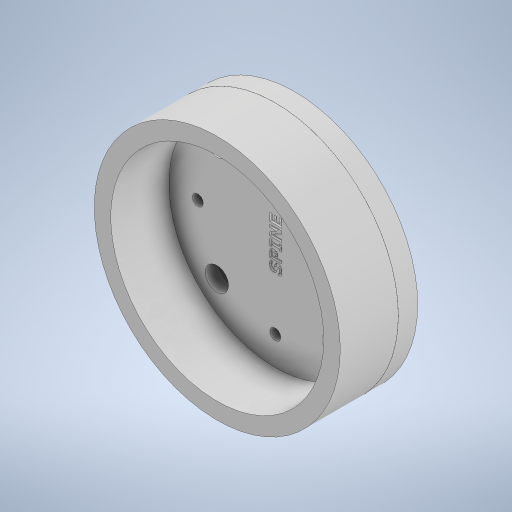
# Autodesk Inventor part: adaptor_spine_transducer_names
Saved by Autodesk Inventor 2024 (Build 280153000, 153)
## iProperties
Created: 2024-05-24
Part Number: adaptor_spine_transducer_names
Material: Generic
Document SubType Name: Modeling
Designer: maint
Density: 1 g/cm^3
Appearance: Default
Author: maint
Autodesk Inventor part; units mm, degrees
ref_plane "YZ Plane" through (0, 0, 0) normal (1, 0, 0) x (0, 1, 0)
ref_plane "XZ Plane" through (0, 0, 0) normal (0, 1, 0) x (-1, 0, 0)
ref_plane "XY Plane" through (0, 0, 0) normal (0, 0, 1) x (1, 0, 0)
sketch "Sketch1" plane through (0, 0, 0) normal (0, 0, 1) x (1, 0, 0)
  line L0 (40, -40) -> (-40, -40)
  line L1 (-40, -40) -> (-40, 40)
  line L2 (-40, 40) -> (40, 40)
  line L3 (40, 40) -> (40, -40)
  line L4 (40, -40) -> (-40, 40) construction
  line L5 (-40, -40) -> (40, 40) construction
  circle A0 centre (0, 0) radius 63.5
  dimension "d0" = 80
  dimension "d72" = 127
  constraints: 12 end point, 2 midpoint, 2 parallel, 2 perpendicular, 1 centre point, 1 coincident, 1 horizontal
  measures "d0" distance of L1.end L2.end
  measures "d72" diameter of A0
extrude "Extrusion1" add sketch "Sketch1" along normal blind 10 contours L0 L1 L2 L3 | A0
sketch "Sketch2" plane through (0, 0, 0) normal (0, 0, -1) x (-1, 0, 0)
  arc A0 (40, 37) -> (37, 40) centre (37, 37) ccw
  line L0 (30.15, -30.15) -> (-30.15, -30.15)
  line L1 (-30.15, -30.15) -> (-30.15, 30.15)
  line L2 (-30.15, 30.15) -> (30.15, 30.15)
  line L3 (30.15, 30.15) -> (30.15, -30.15)
  line L4 (30.15, -30.15) -> (-30.15, 30.15) construction
  line L5 (-30.15, -30.15) -> (30.15, 30.15) construction
  circle A1 centre (-30.15, 30.15) radius 4.75
  circle A2 centre (30.15, 30.15) radius 4.75
  circle A3 centre (30.15, -30.15) radius 4.75
  circle A4 centre (-30.15, -30.15) radius 4.75
  point P0 (0, 0)
  point P1 (39.1213, 39.1213)
  dimension "d32" = 60.3
  dimension "d33" = 9.5
  constraints: 12 end point, 5 centre point, 4 coincident, 3 equal radius, 3 point on circle, 2 midpoint, 2 parallel, 2 perpendicular, 1 horizontal
  measures "d32" distance of L1.end L2.end
  measures "d33" diameter of A2
hole "Hole3" at (30.15, -30.15, 0) at (30.15, 30.15, 0) at (-30.15, 30.15, 0) at (-30.15, -30.15, 0) direction (0, 0, 1) diameter 6.6 end through all
sketch "Sketch3" plane through (0, 0, 0) normal (0, 0, -1) x (-1, 0, 0)
  circle A0 centre (0, 0) radius 40
  circle A1 centre (0, 40) radius 2.5
  circle A2 centre (40, 0) radius 2.5
  circle A3 centre (0, -40) radius 2.5
  circle A4 centre (-40, 0) radius 2.5
  dimension "d12" = 5
  dimension "d60" = 80
  constraints: 5 centre point, 4 point on circle, 3 equal radius
  measures "d12" diameter of A1
  measures "d60" diameter of A0
hole "Hole1" at (40, 0, 0) at (0, 40, 0) at (0, -40, 0) at (-40, 0, 0) direction (0, 0, 1) diameter 5.6 end through all
sketch "Sketch8" plane through (0, 0, 0) normal (0, 0, -1) x (-1, 0, 0)
  circle A0 centre (0, 0) radius 40
  circle A1 centre (0, 40) radius 12.0233
  circle A2 centre (40, 0) radius 12.001
  circle A3 centre (-40, 0) radius 12.185
  circle A4 centre (0, -40) radius 12.001
  dimension "d61" = 80
  constraints: 5 centre point, 4 point on circle, 1 coincident
  measures "d61" diameter of A0
hole "Hole4" at (-40, 0, 0) at (0, 40, 0) at (40, 0, 0) at (0, -40, 0) direction (0, 0, 1) diameter 13 depth 4 tip angle 118
sketch "Sketch10" plane through (0, 0, 10) normal (0, 0, 1) x (1, 0, 0)
  circle A0 centre (30.15, 30.15) radius 3.3 projected
  circle A1 centre (30.15, 30.15) radius 6
  circle A2 centre (-30.15, 30.15) radius 3.3 projected
  circle A3 centre (-30.15, 30.15) radius 6
  circle A4 centre (-30.15, -30.2444) radius 6
  circle A5 centre (30.15, -30.2444) radius 6
  point P0 (0, 0)
  dimension "d63" = 12
  constraints: 4 centre point, 3 equal radius, 2 coincident
  measures "d63" diameter of A1
hole "Hole5" at (-30.15, -30.2444, 10) at (30.15, -30.2444, 10) at (30.15, 30.15, 10) at (-30.15, 30.15, 10) direction (0, 0, -1) diameter 12 depth 7 tip angle 118
sketch "Sketch11" plane through (0, 0, 0) normal (0, 0, -1) x (-1, 0, 0)
  line L0 (2.543, 18.4604) -> (2.543, -5.1802) construction
  line L1 (2.543, -5.1802) -> (11.8674, -5.1802) construction
  line L2 (11.8674, -5.1802) -> (11.8674, 18.4604) construction
  line L3 (11.8674, 18.4604) -> (2.543, 18.4604) construction
  spline S0 degree 2 poles (-3.7943, 15.9443) (-3.7943, 16.6463) (-3.5224, 17.7041) (-3.3246, 18.1589) knots 0 0 0 1 2 2 2
  line L4 (-3.3246, 18.1589) -> (-1.8713, 18.1589)
  line L5 (-1.8713, 18.1589) -> (-1.8713, 18.0205)
  spline S1 degree 2 poles (-1.8713, 18.0205) (-2.2618, 17.5608) (-2.682, 16.4584) (-2.682, 15.9394) knots 0 0 0 1 2 2 2
  spline S2 degree 2 poles (-2.682, 15.9394) (-2.682, 15.8059) (-2.6227, 15.3758) (-2.5634, 15.2473) knots 0 0 0 1 2 2 2
  spline S3 degree 2 poles (-2.5634, 15.2473) (-2.4942, 15.0891) (-2.2421, 14.8667) (-2.0394, 14.8667) knots 0 0 0 1 2 2 2
  spline S4 degree 2 poles (-2.0394, 14.8667) (-1.8071, 14.8667) (-1.5204, 15.2275) (-1.4561, 15.4747) knots 0 0 0 1 2 2 2
  spline S5 degree 2 poles (-1.4561, 15.4747) (-1.3721, 15.7861) (-1.2287, 16.493) (-1.1199, 16.8044) knots 0 0 0 1 2 2 2
  spline S6 degree 2 poles (-1.1199, 16.8044) (-0.8728, 17.5113) (-0.0275, 18.1243) (0.6053, 18.1243) knots 0 0 0 1 2 2 2
  spline S7 degree 2 poles (0.6053, 18.1243) (1.4604, 18.1243) (2.5232, 16.6759) (2.5232, 15.5884) knots 0 0 0 1 2 2 2
  spline S8 degree 2 poles (2.5232, 15.5884) (2.5232, 15.0446) (2.3008, 13.967) (2.113, 13.5419) knots 0 0 0 1 2 2 2
  line L6 (2.113, 13.5419) -> (0.719, 13.5419)
  line L7 (0.719, 13.5419) -> (0.719, 13.6753)
  spline S9 degree 2 poles (0.719, 13.6753) (1.0106, 14.0164) (1.411, 14.9952) (1.411, 15.5093) knots 0 0 0 1 2 2 2
  spline S10 degree 2 poles (1.411, 15.5093) (1.411, 15.712) (1.3517, 16.0283) (1.2726, 16.2063) knots 0 0 0 1 2 2 2
  spline S11 degree 2 poles (1.2726, 16.2063) (1.2083, 16.3497) (0.9513, 16.5573) (0.7931, 16.5573) knots 0 0 0 1 2 2 2
  spline S12 degree 2 poles (0.7931, 16.5573) (0.5558, 16.5573) (0.2839, 16.2261) (0.1752, 15.7515) knots 0 0 0 1 2 2 2
  spline S13 degree 2 poles (0.1752, 15.7515) (0.106, 15.445) (-0.0275, 14.8766) (-0.1412, 14.5503) knots 0 0 0 1 2 2 2
  spline S14 degree 2 poles (-0.1412, 14.5503) (-0.3735, 13.9176) (-1.1447, 13.2997) (-1.7774, 13.2997) knots 0 0 0 1 2 2 2
  spline S15 degree 2 poles (-1.7774, 13.2997) (-2.687, 13.2997) (-3.7943, 14.7283) (-3.7943, 15.9443) knots 0 0 0 1 2 2 2
  line L8 (-3.6855, 12.5137) -> (2.4145, 12.5137)
  line L9 (2.4145, 12.5137) -> (2.4145, 8.391)
  line L10 (2.4145, 8.391) -> (1.2528, 8.391)
  line L11 (1.2528, 8.391) -> (1.2528, 10.9911)
  line L12 (1.2528, 10.9911) -> (0.1801, 10.9911)
  line L13 (0.1801, 10.9911) -> (0.1801, 8.5937)
  line L14 (0.1801, 8.5937) -> (-0.9815, 8.5937)
  line L15 (-0.9815, 8.5937) -> (-0.9815, 10.9911)
  line L16 (-0.9815, 10.9911) -> (-2.5238, 10.9911)
  line L17 (-2.5238, 10.9911) -> (-2.5238, 8.391)
  line L18 (-2.5238, 8.391) -> (-3.6855, 8.391)
  line L19 (-3.6855, 8.391) -> (-3.6855, 12.5137)
  line L20 (-3.6855, 2.1279) -> (-3.6855, 3.601)
  line L21 (-3.6855, 3.601) -> (0.5657, 5.9539)
  line L22 (0.5657, 5.9539) -> (-3.6855, 5.9539)
  line L23 (-3.6855, 5.9539) -> (-3.6855, 7.3529)
  line L24 (-3.6855, 7.3529) -> (2.4145, 7.3529)
  line L25 (2.4145, 7.3529) -> (2.4145, 5.4745)
  line L26 (2.4145, 5.4745) -> (-1.0804, 3.5268)
  line L27 (-1.0804, 3.5268) -> (2.4145, 3.5268)
  line L28 (2.4145, 3.5268) -> (2.4145, 2.1279)
  line L29 (2.4145, 2.1279) -> (-3.6855, 2.1279)
  spline S16 degree 2 poles (-3.7943, -0.9963) (-3.7943, -0.2943) (-3.5224, 0.7635) (-3.3246, 1.2183) knots 0 0 0 1 2 2 2
  line L30 (-3.3246, 1.2183) -> (-1.8713, 1.2183)
  line L31 (-1.8713, 1.2183) -> (-1.8713, 1.0799)
  spline S17 degree 2 poles (-1.8713, 1.0799) (-2.2618, 0.6202) (-2.682, -0.4822) (-2.682, -1.0012) knots 0 0 0 1 2 2 2
  spline S18 degree 2 poles (-2.682, -1.0012) (-2.682, -1.1347) (-2.6227, -1.5648) (-2.5634, -1.6933) knots 0 0 0 1 2 2 2
  spline S19 degree 2 poles (-2.5634, -1.6933) (-2.4942, -1.8515) (-2.2421, -2.0739) (-2.0394, -2.0739) knots 0 0 0 1 2 2 2
  spline S20 degree 2 poles (-2.0394, -2.0739) (-1.8071, -2.0739) (-1.5204, -1.7131) (-1.4561, -1.4659) knots 0 0 0 1 2 2 2
  spline S21 degree 2 poles (-1.4561, -1.4659) (-1.3721, -1.1545) (-1.2287, -0.4476) (-1.1199, -0.1362) knots 0 0 0 1 2 2 2
  spline S22 degree 2 poles (-1.1199, -0.1362) (-0.8728, 0.5707) (-0.0275, 1.1837) (0.6053, 1.1837) knots 0 0 0 1 2 2 2
  spline S23 degree 2 poles (0.6053, 1.1837) (1.4604, 1.1837) (2.5232, -0.2647) (2.5232, -1.3522) knots 0 0 0 1 2 2 2
  spline S24 degree 2 poles (2.5232, -1.3522) (2.5232, -1.896) (2.3008, -2.9736) (2.113, -3.3987) knots 0 0 0 1 2 2 2
  line L32 (2.113, -3.3987) -> (0.719, -3.3987)
  line L33 (0.719, -3.3987) -> (0.719, -3.2653)
  spline S25 degree 2 poles (0.719, -3.2653) (1.0106, -2.9242) (1.411, -1.9454) (1.411, -1.4313) knots 0 0 0 1 2 2 2
  spline S26 degree 2 poles (1.411, -1.4313) (1.411, -1.2286) (1.3517, -0.9123) (1.2726, -0.7343) knots 0 0 0 1 2 2 2
  spline S27 degree 2 poles (1.2726, -0.7343) (1.2083, -0.5909) (0.9513, -0.3833) (0.7931, -0.3833) knots 0 0 0 1 2 2 2
  spline S28 degree 2 poles (0.7931, -0.3833) (0.5558, -0.3833) (0.2839, -0.7145) (0.1752, -1.1891) knots 0 0 0 1 2 2 2
  spline S29 degree 2 poles (0.1752, -1.1891) (0.106, -1.4956) (-0.0275, -2.064) (-0.1412, -2.3903) knots 0 0 0 1 2 2 2
  spline S30 degree 2 poles (-0.1412, -2.3903) (-0.3735, -3.023) (-1.1447, -3.6409) (-1.7774, -3.6409) knots 0 0 0 1 2 2 2
  spline S31 degree 2 poles (-1.7774, -3.6409) (-2.687, -3.6409) (-3.7943, -2.2123) (-3.7943, -0.9963) knots 0 0 0 1 2 2 2
  spline S32 degree 2 poles (-0.6355, -9.9782) (-2.1185, -9.9782) (-3.814, -8.3964) (-3.814, -7.0221) knots 0 0 0 1 2 2 2
  spline S33 degree 2 poles (-3.814, -7.0221) (-3.814, -5.643) (-2.0987, -4.071) (-0.6355, -4.071) knots 0 0 0 1 2 2 2
  spline S34 degree 2 poles (-0.6355, -4.071) (0.8326, -4.071) (2.543, -5.643) (2.543, -7.0221) knots 0 0 0 1 2 2 2
  spline S35 degree 2 poles (2.543, -7.0221) (2.543, -8.3964) (0.8425, -9.9782) (-0.6355, -9.9782) knots 0 0 0 1 2 2 2
  spline S36 degree 2 poles (-0.6355, -8.3964) (-0.0868, -8.3964) (0.6794, -8.1739) (0.9216, -7.9811) knots 0 0 0 1 2 2 2
  spline S37 degree 2 poles (0.9216, -7.9811) (1.1737, -7.7884) (1.3912, -7.294) (1.3912, -7.0271) knots 0 0 0 1 2 2 2
  spline S38 degree 2 poles (1.3912, -7.0271) (1.3912, -6.7453) (1.1886, -6.2856) (0.9315, -6.073) knots 0 0 0 1 2 2 2
  spline S39 degree 2 poles (0.9315, -6.073) (0.6942, -5.8852) (-0.0917, -5.6529) (-0.6355, -5.6529) knots 0 0 0 1 2 2 2
  spline S40 degree 2 poles (-0.6355, -5.6529) (-1.199, -5.6529) (-1.9405, -5.8753) (-2.1926, -6.0681) knots 0 0 0 1 2 2 2
  spline S41 degree 2 poles (-2.1926, -6.0681) (-2.4447, -6.2609) (-2.6622, -6.7602) (-2.6622, -7.0271) knots 0 0 0 1 2 2 2
  spline S42 degree 2 poles (-2.6622, -7.0271) (-2.6622, -7.299) (-2.4299, -7.8032) (-2.1828, -7.9861) knots 0 0 0 1 2 2 2
  spline S43 degree 2 poles (-2.1828, -7.9861) (-1.9158, -8.1838) (-1.2089, -8.3964) (-0.6355, -8.3964) knots 0 0 0 1 2 2 2
  line L34 (-3.6855, -16.5231) -> (-3.6855, -14.6595)
  line L35 (-3.6855, -14.6595) -> (-1.4462, -12.964)
  line L36 (-1.4462, -12.964) -> (-1.4462, -12.4103)
  line L37 (-1.4462, -12.4103) -> (-3.6855, -12.4103)
  line L38 (-3.6855, -12.4103) -> (-3.6855, -10.8878)
  line L39 (-3.6855, -10.8878) -> (2.4145, -10.8878)
  line L40 (2.4145, -10.8878) -> (2.4145, -13.3396)
  spline S44 degree 2 poles (2.4145, -13.3396) (2.4145, -13.8488) (2.286, -14.6002) (2.0882, -14.9215) knots 0 0 0 1 2 2 2
  spline S45 degree 2 poles (2.0882, -14.9215) (1.8806, -15.2478) (1.2331, -15.6333) (0.7387, -15.6333) knots 0 0 0 1 2 2 2
  spline S46 degree 2 poles (0.7387, -15.6333) (0.0417, -15.6333) (-0.8332, -15.0006) (-1.0903, -14.4717) knots 0 0 0 1 2 2 2
  line L41 (-1.0903, -14.4717) -> (-3.6855, -16.5231)
  spline S47 degree 2 poles (0.5459, -14.0614) (0.7783, -14.0614) (1.1095, -13.8834) (1.1984, -13.6807) knots 0 0 0 1 2 2 2
  spline S48 degree 2 poles (1.1984, -13.6807) (1.2578, -13.5374) (1.2924, -13.1864) (1.2924, -12.9244) knots 0 0 0 1 2 2 2
  line L42 (1.2924, -12.9244) -> (1.2924, -12.4103)
  line L43 (1.2924, -12.4103) -> (-0.3488, -12.4103)
  line L44 (-0.3488, -12.4103) -> (-0.3488, -12.8503)
  spline S49 degree 2 poles (-0.3488, -12.8503) (-0.3488, -13.1666) (-0.2697, -13.6165) (-0.1461, -13.7697) knots 0 0 0 1 2 2 2
  spline S50 degree 2 poles (-0.1461, -13.7697) (-0.0275, -13.918) (0.2889, -14.0614) (0.5459, -14.0614) knots 0 0 0 1 2 2 2
  point P0 (0, 0)
  constraints: 2 other
extrude "Extrusion5" cut sketch "Sketch11" against normal blind 1
sketch "Sketch12" plane through (0, 0, 10) normal (0, 0, 1) x (1, 0, 0)
  line L0 (-2.9198, -12.9035) -> (-2.9198, 8.4327) construction
  line L1 (-2.9198, 8.4327) -> (-6.222, 8.4327) construction
  line L2 (-6.222, 8.4327) -> (-6.222, -12.9035) construction
  line L3 (-6.222, -12.9035) -> (-2.9198, -12.9035) construction
  spline S0 degree 2 poles (3.3977, -10.3873) (3.3977, -11.0893) (3.1259, -12.1471) (2.9281, -12.6019) knots 0 0 0 1 2 2 2
  line L4 (2.9281, -12.6019) -> (1.4748, -12.6019)
  line L5 (1.4748, -12.6019) -> (1.4748, -12.4635)
  spline S1 degree 2 poles (1.4748, -12.4635) (1.8653, -12.0038) (2.2855, -10.9014) (2.2855, -10.3824) knots 0 0 0 1 2 2 2
  spline S2 degree 2 poles (2.2855, -10.3824) (2.2855, -10.2489) (2.2262, -9.8189) (2.1669, -9.6903) knots 0 0 0 1 2 2 2
  spline S3 degree 2 poles (2.1669, -9.6903) (2.0977, -9.5322) (1.8456, -9.3097) (1.6429, -9.3097) knots 0 0 0 1 2 2 2
  spline S4 degree 2 poles (1.6429, -9.3097) (1.4105, -9.3097) (1.1238, -9.6706) (1.0596, -9.9177) knots 0 0 0 1 2 2 2
  spline S5 degree 2 poles (1.0596, -9.9177) (0.9755, -10.2292) (0.8322, -10.936) (0.7234, -11.2475) knots 0 0 0 1 2 2 2
  spline S6 degree 2 poles (0.7234, -11.2475) (0.4763, -11.9544) (-0.369, -12.5673) (-1.0018, -12.5673) knots 0 0 0 1 2 2 2
  spline S7 degree 2 poles (-1.0018, -12.5673) (-1.857, -12.5673) (-2.9198, -11.1189) (-2.9198, -10.0314) knots 0 0 0 1 2 2 2
  spline S8 degree 2 poles (-2.9198, -10.0314) (-2.9198, -9.4877) (-2.6973, -8.41) (-2.5095, -7.9849) knots 0 0 0 1 2 2 2
  line L6 (-2.5095, -7.9849) -> (-1.1155, -7.9849)
  line L7 (-1.1155, -7.9849) -> (-1.1155, -8.1184)
  spline S9 degree 2 poles (-1.1155, -8.1184) (-1.4071, -8.4595) (-1.8075, -9.4382) (-1.8075, -9.9523) knots 0 0 0 1 2 2 2
  spline S10 degree 2 poles (-1.8075, -9.9523) (-1.8075, -10.155) (-1.7482, -10.4714) (-1.6691, -10.6493) knots 0 0 0 1 2 2 2
  spline S11 degree 2 poles (-1.6691, -10.6493) (-1.6049, -10.7927) (-1.3478, -11.0003) (-1.1896, -11.0003) knots 0 0 0 1 2 2 2
  spline S12 degree 2 poles (-1.1896, -11.0003) (-0.9523, -11.0003) (-0.6805, -10.6691) (-0.5717, -10.1946) knots 0 0 0 1 2 2 2
  spline S13 degree 2 poles (-0.5717, -10.1946) (-0.5025, -9.8881) (-0.369, -9.3196) (-0.2553, -8.9933) knots 0 0 0 1 2 2 2
  spline S14 degree 2 poles (-0.2553, -8.9933) (-0.023, -8.3606) (0.7481, -7.7427) (1.3809, -7.7427) knots 0 0 0 1 2 2 2
  spline S15 degree 2 poles (1.3809, -7.7427) (2.2904, -7.7427) (3.3977, -9.1713) (3.3977, -10.3873) knots 0 0 0 1 2 2 2
  spline S16 degree 2 poles (-0.8881, -2.2655) (-0.463, -2.2655) (0.3082, -2.5374) (0.5652, -2.7895) knots 0 0 0 1 2 2 2
  spline S17 degree 2 poles (0.5652, -2.7895) (0.7284, -2.9428) (0.9953, -3.3185) (1.0892, -3.5409) knots 0 0 0 1 2 2 2
  spline S18 degree 2 poles (1.0892, -3.5409) (1.1832, -3.7683) (1.2919, -4.2972) (1.2919, -4.6235) knots 0 0 0 1 2 2 2
  line L8 (1.2919, -4.6235) -> (1.2919, -5.4243)
  line L9 (1.2919, -5.4243) -> (3.289, -5.4243)
  line L10 (3.289, -5.4243) -> (3.289, -6.9567)
  line L11 (3.289, -6.9567) -> (-2.811, -6.9567)
  line L12 (-2.811, -6.9567) -> (-2.811, -4.5889)
  spline S19 degree 2 poles (-2.811, -4.5889) (-2.811, -4.0649) (-2.6182, -3.2987) (-2.4106, -2.9873) knots 0 0 0 1 2 2 2
  spline S20 degree 2 poles (-2.4106, -2.9873) (-2.1783, -2.6412) (-1.417, -2.2655) (-0.8881, -2.2655) knots 0 0 0 1 2 2 2
  spline S21 degree 2 poles (-0.8485, -3.8375) (-1.1105, -3.8375) (-1.4813, -4.0847) (-1.5505, -4.2527) knots 0 0 0 1 2 2 2
  spline S22 degree 2 poles (-1.5505, -4.2527) (-1.6444, -4.4702) (-1.6741, -4.8657) (-1.6741, -5.2068) knots 0 0 0 1 2 2 2
  line L13 (-1.6741, -5.2068) -> (-1.6741, -5.4243)
  line L14 (-1.6741, -5.4243) -> (0.155, -5.4243)
  line L15 (0.155, -5.4243) -> (0.155, -5.3155)
  spline S23 degree 2 poles (0.155, -5.3155) (0.155, -5.103) (0.1451, -4.7174) (0.1204, -4.574) knots 0 0 0 1 2 2 2
  spline S24 degree 2 poles (0.1204, -4.574) (0.1006, -4.4505) (-0.0181, -4.1786) (-0.0922, -4.1044) knots 0 0 0 1 2 2 2
  spline S25 degree 2 poles (-0.0922, -4.1044) (-0.2405, -3.9463) (-0.5717, -3.8375) (-0.8485, -3.8375) knots 0 0 0 1 2 2 2
  line L16 (3.289, 1.5902) -> (3.289, -1.6921)
  line L17 (3.289, -1.6921) -> (2.2262, -1.6921)
  line L18 (2.2262, -1.6921) -> (2.2262, -0.8172)
  line L19 (2.2262, -0.8172) -> (-1.7482, -0.8172)
  line L20 (-1.7482, -0.8172) -> (-1.7482, -1.6921)
  line L21 (-1.7482, -1.6921) -> (-2.811, -1.6921)
  line L22 (-2.811, -1.6921) -> (-2.811, 1.5902)
  line L23 (-2.811, 1.5902) -> (-1.7482, 1.5902)
  line L24 (-1.7482, 1.5902) -> (-1.7482, 0.7153)
  line L25 (-1.7482, 0.7153) -> (2.2262, 0.7153)
  line L26 (2.2262, 0.7153) -> (2.2262, 1.5902)
  line L27 (2.2262, 1.5902) -> (3.289, 1.5902)
  line L28 (3.289, 7.8336) -> (3.289, 6.3605)
  line L29 (3.289, 6.3605) -> (-0.9622, 4.0075)
  line L30 (-0.9622, 4.0075) -> (3.289, 4.0075)
  line L31 (3.289, 4.0075) -> (3.289, 2.6085)
  line L32 (3.289, 2.6085) -> (-2.811, 2.6085)
  line L33 (-2.811, 2.6085) -> (-2.811, 4.487)
  line L34 (-2.811, 4.487) -> (0.6839, 6.4346)
  line L35 (0.6839, 6.4346) -> (-2.811, 6.4346)
  line L36 (-2.811, 6.4346) -> (-2.811, 7.8336)
  line L37 (-2.811, 7.8336) -> (3.289, 7.8336)
  line L38 (3.289, 9.0743) -> (-2.811, 9.0743)
  line L39 (-2.811, 9.0743) -> (-2.811, 13.197)
  line L40 (-2.811, 13.197) -> (-1.6493, 13.197)
  line L41 (-1.6493, 13.197) -> (-1.6493, 10.5969)
  line L42 (-1.6493, 10.5969) -> (-0.5767, 10.5969)
  line L43 (-0.5767, 10.5969) -> (-0.5767, 12.9943)
  line L44 (-0.5767, 12.9943) -> (0.585, 12.9943)
  line L45 (0.585, 12.9943) -> (0.585, 10.5969)
  line L46 (0.585, 10.5969) -> (2.1273, 10.5969)
  line L47 (2.1273, 10.5969) -> (2.1273, 13.197)
  line L48 (2.1273, 13.197) -> (3.289, 13.197)
  line L49 (3.289, 13.197) -> (3.289, 9.0743)
  point P0 (0, 0)
  constraints: 2 other
extrude "Extrusion6" cut sketch "Sketch12" against normal blind 1
sketch "Sketch13" plane through (0, 0, 0) normal (0, 0, -1) x (-1, 0, 0)
  line L0 (-52.0548, -4.6689) -> (-55.7273, -0.7894) construction
  line L1 (-55.7273, -0.7894) -> (-50.7734, 3.9002) construction
  line L2 (-50.7734, 3.9002) -> (-47.1009, 0.0207) construction
  line L3 (-47.1009, 0.0207) -> (-52.0548, -4.6689) construction
  line L4 (-52.9473, 3.7508) -> (-47.7576, 8.6636) construction
  line L5 (-47.7576, 8.6636) -> (-44.0585, 4.7561) construction
  line L6 (-44.0585, 4.7561) -> (-49.2482, -0.1567) construction
  line L7 (-49.2482, -0.1567) -> (-52.9473, 3.7508) construction
  line L8 (-50.1822, -1.3003) -> (-50.1822, -4.3034) construction
  line L9 (-50.1822, -4.3034) -> (-51.9606, -4.3034) construction
  line L10 (-51.9606, -4.3034) -> (-51.9606, -1.3003) construction
  line L11 (-51.9606, -1.3003) -> (-50.1822, -1.3003) construction
  line L12 (-46.238, 11.5483) -> (-46.238, 9.2121) construction
  line L13 (-46.238, 9.2121) -> (-50.3267, 9.2121) construction
  line L14 (-50.3267, 9.2121) -> (-50.3267, 11.5483) construction
  line L15 (-50.3267, 11.5483) -> (-46.238, 11.5483) construction
  line L16 (-52.7292, 1.3372) -> (-52.7508, 0.1538)
  line L17 (-52.7508, 0.1538) -> (-48.1785, 0.0367)
  line L18 (-48.1785, 0.0367) -> (-48.1793, -0.4874)
  line L19 (-48.1793, -0.4874) -> (-52.7621, -0.3591)
  line L20 (-52.7621, -0.3591) -> (-52.7995, -1.5257)
  line L21 (-52.7995, -1.5257) -> (-56.5565, 0.0029)
  line L22 (-56.5565, 0.0029) -> (-52.7292, 1.3372)
  line L23 (-46.9412, 4.4253) -> (-48.1246, 4.4468)
  line L24 (-48.1246, 4.4468) -> (-48.2418, -0.1255)
  line L25 (-48.2418, -0.1255) -> (-48.7658, -0.1247)
  line L26 (-48.7658, -0.1247) -> (-48.6375, 4.4582)
  line L27 (-48.6375, 4.4582) -> (-49.8041, 4.4956)
  line L28 (-49.8041, 4.4956) -> (-48.2755, 8.2526)
  line L29 (-48.2755, 8.2526) -> (-46.9412, 4.4253)
  line L30 (-49.408, 8.5376) -> (-49.408, 9.4573)
  line L31 (-49.408, 9.4573) -> (-48.3985, 10.0687)
  line L32 (-48.3985, 10.0687) -> (-49.408, 10.6929)
  line L33 (-49.408, 10.6929) -> (-49.408, 11.574)
  line L34 (-49.408, 11.574) -> (-47.8128, 10.5439)
  line L35 (-47.8128, 10.5439) -> (-46.238, 11.5329)
  line L36 (-46.238, 11.5329) -> (-46.238, 10.6133)
  line L37 (-46.238, 10.6133) -> (-47.1962, 10.0404)
  line L38 (-47.1962, 10.0404) -> (-46.238, 9.4521)
  line L39 (-46.238, 9.4521) -> (-46.238, 8.571)
  line L40 (-46.238, 8.571) -> (-47.7794, 9.5652)
  line L41 (-47.7794, 9.5652) -> (-49.408, 8.5376)
  line L42 (-50.1822, -4.2648) -> (-52.0292, -3.1705)
  line L43 (-52.0292, -3.1705) -> (-53.3522, -3.1705)
  line L44 (-53.3522, -3.1705) -> (-53.3522, -2.3741)
  line L45 (-53.3522, -2.3741) -> (-52.0678, -2.3741)
  line L46 (-52.0678, -2.3741) -> (-50.1822, -1.2618)
  line L47 (-50.1822, -1.2618) -> (-50.1822, -2.1686)
  line L48 (-50.1822, -2.1686) -> (-51.3125, -2.7877)
  line L49 (-51.3125, -2.7877) -> (-50.1822, -3.3863)
  line L50 (-50.1822, -3.3863) -> (-50.1822, -4.2648)
  point P0 (0, 0)
  constraints: 8 other
extrude "Extrusion7" cut sketch "Sketch13" against normal blind 1
sketch "Sketch16" plane through (0, 0, 10) normal (0, 0, 1) x (1, 0, 0)
  circle A0 centre (0, 0) radius 55
  circle A1 centre (0, 0) radius 63.535
  dimension "d81" = 110
  constraints: 2 centre point, 2 coincident
  measures "d81" diameter of A0
extrude "Extrusion9" add sketch "Sketch16" along normal blind 30
body "Solid1"
